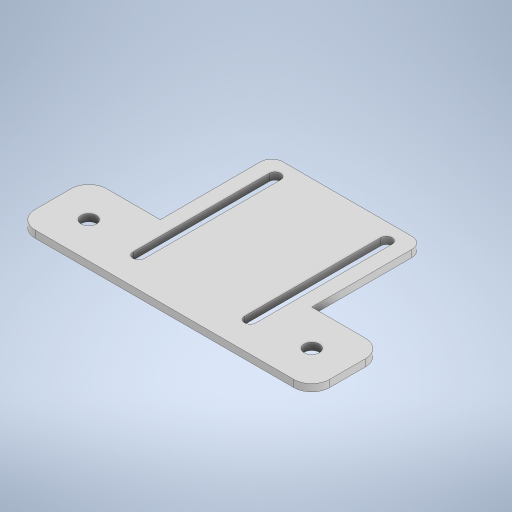
# Autodesk Inventor part: Motor Attachment Small 3.0
Saved by Autodesk Inventor 2024 (Build 280153000, 153)
## iProperties
Created: 2023-10-21
Part Number: Motor Attachment Small 3.0
Material: Generic
Document SubType Name: Modeling
Designer: olson
Density: 1 g/cm^3
Appearance: Default
Author: olson
Autodesk Inventor part; units mm, degrees
ref_plane "YZ Plane" through (0, 0, 0) normal (1, 0, 0) x (0, 1, 0)
ref_plane "XZ Plane" through (0, 0, 0) normal (0, 1, 0) x (-1, 0, 0)
ref_plane "XY Plane" through (0, 0, 0) normal (0, 0, 1) x (1, 0, 0)
sketch "Sketch1" plane through (0, 0, 0) normal (0, 1, 0) x (-1, 0, 0)
  line L0 (0, 0) -> (-42.4, 0)
  line L1 (-42.4, -20) -> (-42.4, -51.2)
  line L2 (-42.4, -51.2) -> (0, -51.2)
  line L3 (0, -51.2) -> (0, -20)
  line L4 (-21.2, 0) -> (-6.45, 0)
  line L5 (-6.45, 0) -> (-28.15, 0)
  line L6 (-21.2, 0) -> (0.55, 0)
  line L7 (0.55, 0) -> (-30.65, 0)
  line L8 (-21.2, 0) -> (-5.6, 0)
  line L9 (-5.6, 0) -> (-36.8, 0)
  arc A0 (-35.2, -8.4) -> (-38.4, -8.4) centre (-36.8, -8.4) ccw
  arc A1 (-38.4, -46.5) -> (-35.2, -46.5) centre (-36.8, -46.5) ccw
  arc A2 (-4, -8.4) -> (-7.2, -8.4) centre (-5.6, -8.4) ccw
  arc A3 (-7.2, -46.5) -> (-4, -46.5) centre (-5.6, -46.5) ccw
  line L10 (0, 0) -> (0, -20)
  line L11 (0, -20) -> (20, -20)
  line L12 (20, -20) -> (20, 0)
  line L13 (20, 0) -> (0, 0)
  line L14 (-42.4, -20) -> (-62.4, -20)
  line L15 (-62.4, -20) -> (-62.4, 0)
  line L16 (-62.4, 0) -> (-42.4, 0)
  line L17 (-4, -46.5) -> (-4, -8.4)
  line L18 (-7.2, -8.4) -> (-7.2, -46.5)
  line L19 (-35.2, -46.5) -> (-35.2, -8.4)
  line L20 (-38.4, -8.4) -> (-38.4, -46.5)
  dimension "d0" = 42.4
  dimension "d1" = 51.2
  dimension "d41" = 15.6
  dimension "d42" = 31.2
  dimension "d50" = 3.2
  dimension "d56" = 3.2
  dimension "d57" = 3.2
  dimension "d63" = 3.2
  dimension "d67" = 8.4
  dimension "d77" = 8.4
  dimension "d81" = 20
  dimension "d82" = 20
  dimension "d83" = 20
  constraints: 42 end point, 9 point on line, 8 point on circle, 6 perpendicular, 6 tangent, 4 centre point, 2 parallel, 1 horizontal, 1 midpoint
  measures "d0" distance of L2.end L1.end
  measures "d1" distance of L1.end L0.end
  measures "d41" distance of L4.start L8.end
  measures "d42" distance of L8.end L9.end
  measures "d50" diameter of A0
  measures "d56" diameter of A1
  measures "d57" diameter of A2
  measures "d63" diameter of A3
  measures "d67" distance of L8.end A2.centre
  measures "d77" distance of L9.end A0.centre
  measures "d81" distance of L3.end L0.start
  measures "d82" distance of L3.end L11.end
  measures "d83" distance of L1.start L14.end
extrude "Extrusion3" add sketch "Sketch1" along normal blind 2
fillet "Fillet2" radius 3.175 2 edges at (0, 1, -51.2) (42.4, 1, -51.2)
sketch "Sketch2" plane through (0, 2, 0) normal (0, 1, 0) x (1, 0, 0)
  circle A0 centre (-10, 10) radius 2.125
  line L0 (-20, 0) -> (62.4, 0) projected
  line L1 (38.17, 0) -> (48.17, 0)
  line L2 (62.4, 0) -> (52.4, 0)
  line L3 (-20, 0) -> (62.4, 0) projected
  line L4 (52.4, 0) -> (52.4, 10)
  circle A1 centre (52.4, 10) radius 2.125
  point P0 (0, 0)
  dimension "d85" = 4.25
  dimension "d92" = 10
  dimension "d93" = 10
  dimension "d94" = 4.25
  constraints: 6 end point, 3 point on line, 2 centre point, 1 coincident, 1 vertical
  measures "d85" diameter of A0
  measures "d92" distance of L0.end L2.end
  measures "d93" distance of L2.end L4.end
  measures "d94" diameter of A1
extrude "Extrusion4" cut sketch "Sketch2" against normal blind 2
fillet "Fillet3" radius 5 4 edges at (62.4, 1, -20) (62.4, 1, 0) (-20, 1, 0) (-20, 1, -20)
body "Solid3"
